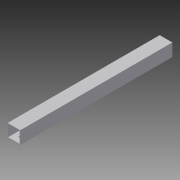
# Autodesk Inventor part: Ram
Saved by Autodesk Inventor 2013 (Build 170138000, 138)
## iProperties
Created: 2013-01-27
Part Number: Ram
Material: Generic
Document SubType Name: Modeling
Designer: carneeki
Density: 1 g/cm^3
Author: carneeki
Autodesk Inventor part; units mm, degrees
ref_plane "YZ Plane" through (0, 0, 0) normal (1, 0, 0) x (0, 1, 0)
ref_plane "XZ Plane" through (0, 0, 0) normal (0, 1, 0) x (-1, 0, 0)
ref_plane "XY Plane" through (0, 0, 0) normal (0, 0, 1) x (1, 0, 0)
sketch "Sketch1" plane through (0, 0, 0) normal (0, 0, 1) x (1, 0, 0)
  line L0 (-12.7, 12.7) -> (12.7, 12.7)
  line L1 (12.7, 12.7) -> (12.7, -12.7)
  line L2 (12.7, -12.7) -> (-12.7, -12.7)
  line L3 (-12.7, -12.7) -> (-12.7, 12.7)
  line L4 (-11.9488, 11.7) -> (11.7, 11.7)
  line L5 (11.7, 11.7) -> (11.7, -11.7)
  line L6 (11.7, -11.7) -> (-11.9488, -11.7)
  line L7 (-11.9488, -11.7) -> (-11.9488, 11.7)
  point P0 (0, 0)
  dimension "d0" = 25.4
  dimension "d1" = 25.4
  dimension "d2" = 12.7
  dimension "d3" = 12.7
  dimension "d4" = 1
  dimension "d5" = 24.6488
  dimension "d6" = 1
  dimension "d8" = 1
  constraints: 16 end point, 4 parallel, 2 horizontal, 2 perpendicular
  measures "d0" distance between parallel lines of L1 L3
  measures "d1" distance between parallel lines of L0 L2
  measures "d2" distance from line of point (0, 0) L1
  measures "d3" distance from line of point (0, 0) L0
  measures "d4" distance between parallel lines of L5 L1
  measures "d5" distance between parallel lines of L7 L1
  measures "d6" distance between parallel lines of L4 L0
  measures "d8" distance between parallel lines of L2 L6
extrude "Extrusion1" add sketch "Sketch1" against normal blind 304.8
sketch "Sketch2" plane through (-12.7, -12.7, 0) normal (0, -1, 0) x (1, 0, 0)
  line L0 (25.4, 0) -> (25.4, -304.8) projected
  circle A0 centre (12.7, -114.2979) radius 2.5908
  circle A1 centre (12.7, -12.6979) radius 2.5908
  point P0 (12.7, 0)
  dimension "d11" = 5.1816
  dimension "d13" = 12.7
  dimension "d21" = 5.1816
  dimension "d22" = 12.6979
  dimension "d23" = 101.6
  constraints: 2 centre point, 1 vertical alignment
  measures "d11" diameter of A0
  measures "d13" distance from line of L0 A0.centre
  measures "d21" diameter of A1
  measures "d22" distance of point (12.7, 0) A1.centre
  measures "d23" distance of A0.centre A1.centre
hole "Hole1" at (0, -12.7, -114.2979) at (0, -12.7, -12.6979) direction (0, 1, 0) diameter 5.1816 depth 3 tip angle 118
equation "\"d8\" = d4"
body "Solid1"
